holder (Autodesk Fusion 360 design; units mm, degrees)
Autodesk Fusion 360 part; units mm, degrees
sketch "Sketch1" plane through (0, 0, 0) normal (0, 1, 0) x (1, 0, 0)
  line L0 (0, 0) -> (16, 0)
  line L1 (16, -10) -> (0, -10)
  line L2 (0, -10) -> (0, 0)
  line L3 (1.5, -8.5) -> (14.5, -8.5)
  line L4 (14.5, -1.5) -> (1.5, -1.5)
  line L5 (1.5, -1.5) -> (1.5, -8.5)
  line L6 (14.5, -7.5) -> (16, -7.5)
  line L7 (16, -2.5) -> (14.5, -2.5)
  line L8 (16, 0) -> (16, -2.5)
  line L9 (16, -7.5) -> (16, -10)
  line L10 (14.5, -8.5) -> (14.5, -7.5)
  line L11 (14.5, -2.5) -> (14.5, -1.5)
  line L12 (0, -10) -> (16, -10)
  line L13 (16, -10) -> (16, 0)
  line L14 (16, 0) -> (0, 0)
  line L15 (0, 0) -> (0, -10)
  dimension "d2" = 1.5
  dimension "d3" = 1.5
  dimension "d4" = 1.5
  dimension "d5" = 1.5
  dimension "d7" = 1
  dimension "d8" = 1
  dimension "d9" = 13
  dimension "d10" = 10
  constraint horizontal L0
  constraint vertical L8
  constraint horizontal L1
  constraint vertical L2
  constraint coincident L0.start L2.end
  constraint horizontal L3
  constraint vertical L10
  constraint horizontal L4
  constraint vertical L5
  constraint coincident L6.end L8
  constraint perpendicular L6 L8
  constraint coincident L7.end L10
  constraint perpendicular L7 L10
  constraint collinear L8 L9
  constraint collinear L10 L11
  constraint horizontal L12
  constraint vertical L13
  constraint horizontal L14
  constraint vertical L15
  measures "d2" distance of L2 L5
  measures "d3" distance of L8 L10
  measures "d4" distance of L0 L4
  measures "d5" distance of L1 L3
  measures "d7" distance of L3 L6
  measures "d8" distance of L4 L7
  measures "d9" distance of L3.start L3.end
  measures "d10" distance of L0.start L1.end
extrude "Extrude1" add sketch "Sketch1" along normal blind 1
extrude "Extrude2" add sketch "Sketch1" against normal blind 1.6 contours L0 L1 L2 L3 L4 L5 L6 L7 L8 L9 L10 L11 L12 L13 L14 L15
fillet "Fillet1" radius 0.5 8 edges at (8, 1, 10) (0, 1, 5) (8, 1, 0) (16, 1, 5) (16, -0.3, 0) (0, -0.3, 0) (0, -0.3, 10) (16, -0.3, 10)
